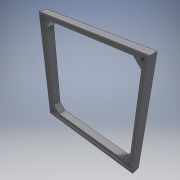
# Autodesk Inventor part: Cougar_Base
Saved by Autodesk Inventor 2018 (Build 220112000, 112)
## iProperties
Created: 2020-04-11
Part Number: Cougar_Base
Material: Všeobecné
Document SubType Name: Modeling
Designer: Jozko Mrkvicka
Density: 1 g/cm^3
Appearance: Výchozí
Author: Jozko Mrkvicka
Autodesk Inventor part; units mm, degrees
ref_plane "YZ Plane" through (0, 0, 0) normal (1, 0, 0) x (0, 1, 0)
ref_plane "XZ Plane" through (0, 0, 0) normal (0, 1, 0) x (-1, 0, 0)
ref_plane "XY Plane" through (0, 0, 0) normal (0, 0, 1) x (1, 0, 0)
sketch "Náčrt1" plane through (0, 0, 0) normal (0, 1, 0) x (-1, 0, 0)
  line L0 (0, 0) -> (178, 0)
  line L1 (178, 0) -> (178, 178)
  line L2 (178, 178) -> (0, 178)
  line L3 (0, 178) -> (0, 0)
  circle A0 centre (9, 9) radius 2
  circle A1 centre (169, 169) radius 2
  circle A2 centre (9, 169) radius 2
  circle A3 centre (169, 9) radius 2
  line L4 (163, 163) -> (157, 169)
  line L5 (163, 15) -> (169, 21)
  line L6 (21, 9) -> (157, 9)
  line L7 (15, 15) -> (21, 9)
  line L8 (15, 15) -> (9, 21)
  line L9 (169, 21) -> (157, 9)
  line L10 (21, 169) -> (9, 157)
  line L11 (9, 157) -> (9, 21)
  line L12 (157, 169) -> (21, 169)
  line L13 (169, 21) -> (169, 157)
  line L14 (163, 163) -> (169, 157)
  dimension "d0" = 178
  dimension "d1" = 178
  dimension "d37" = 9
  dimension "d38" = 9
  constraints: 30 end point, 4 centre point, 4 parallel, 2 horizontal, 2 horizontal alignment, 2 perpendicular, 2 vertical alignment
  measures "d0" distance between parallel lines of L1 L3
  measures "d1" distance between parallel lines of L2 L0
  measures "d37" horizontal distance of L2.end A2.centre
  measures "d38" distance from line of L3 A2.centre
extrude "Vysunutí1" add sketch "Náčrt1" against normal blind 10
sketch "Náčrt2" plane through (0, -10, 0) normal (0, -1, 0) x (1, 0, 0)
  line L0 (-3, 3) -> (-175, 3)
  line L1 (-175, 3) -> (-175, 175)
  line L2 (-175, 175) -> (-3, 175)
  line L3 (-3, 175) -> (-3, 3)
  line L4 (-178, 0) -> (0, 0) projected
  line L5 (0, 0) -> (0, 178) projected
  line L6 (-178, 0) -> (0, 0)
  line L7 (0, 0) -> (0, 178)
  line L8 (0, 178) -> (-178, 178)
  line L9 (-178, 178) -> (-178, 0)
  dimension "d68" = 172
  dimension "d69" = 172
  constraints: 16 end point, 4 parallel, 2 horizontal, 2 perpendicular
  measures "d68" distance of L1.end L2.end
  measures "d69" distance of L0.end L1.end
extrude "Vysunutí2" add sketch "Náčrt2" along normal blind 3
sketch "Náčrt3" plane through (0, 0, 0) normal (0, 1, 0) x (1, 0, 0)
  line L0 (-3, -3) -> (-175, -3)
  line L1 (-175, -3) -> (-175, -175)
  line L2 (-175, -175) -> (-3, -175)
  line L3 (-3, -175) -> (-3, -3)
  line L4 (-169, -21) -> (-157, -9) projected
  line L5 (-157, -9) -> (-169, -21)
  line L6 (-169, -21) -> (-169, -157)
  line L7 (-175, -175) -> (-175, -3) projected
  line L8 (-169, -157) -> (-157, -169)
  line L9 (-21, -169) -> (-157, -169) projected
  line L10 (-157, -169) -> (-21, -169)
  line L11 (-9, -157) -> (-9, -21) projected
  line L12 (-21, -169) -> (-9, -157)
  line L13 (-21, -9) -> (-9, -21) projected
  line L14 (-9, -157) -> (-9, -21)
  line L15 (-9, -21) -> (-21, -9)
  line L16 (-157, -9) -> (-21, -9) projected
  line L17 (-21, -9) -> (-157, -9)
  circle A0 centre (-9, -9) radius 2
  circle A1 centre (-9, -169) radius 2 projected
  circle A2 centre (-9, -169) radius 2
  circle A3 centre (-169, -9) radius 2
  circle A4 centre (-169, -169) radius 2
  constraints: 24 end point, 4 centre point, 4 collinear, 4 parallel, 3 perpendicular, 1 coincident, 1 horizontal
extrude "Vysunutí4" add sketch "Náčrt3" along normal blind 3
